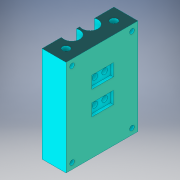
# Autodesk Inventor part: PowerPlugBlock
Saved by Autodesk Inventor 2019 (Build 230136000, 136)
## iProperties
Created: 2020-04-21
Part Number: PowerPlugBlock
Material: Generic
Document SubType Name: Modeling
Designer: james
Density: 1 g/cm^3
Appearance: Default(3)
Author: james
Autodesk Inventor part; units mm, degrees
ref_plane "YZ Plane" through (0, 0, 0) normal (1, 0, 0) x (0, 1, 0)
ref_plane "XZ Plane" through (0, 0, 0) normal (0, 1, 0) x (-1, 0, 0)
ref_plane "XY Plane" through (0, 0, 0) normal (0, 0, 1) x (1, 0, 0)
sketch "Sketch1" plane through (0, 0, 0) normal (0, 1, 0) x (-1, 0, 0)
  line L0 (7.4947, 23.2617) -> (-5.2053, 23.2617)
  line L1 (-5.2053, 23.2617) -> (-5.2053, -14.8383)
  line L2 (-5.2053, -14.8383) -> (7.4947, -14.8383)
  line L3 (7.4947, -14.8383) -> (7.4947, 23.2617)
  point P0 (0, 0)
  dimension "d0" = 38.1
  dimension "d1" = 12.7
  constraints: 8 end point, 2 parallel, 1 horizontal, 1 perpendicular
  measures "d0" distance of L0.end L1.end
  measures "d1" distance of L0.start L0.end
extrude "Extrusion1" add sketch "Sketch1" along normal blind 50.8
sketch "Sketch2" plane through (5.2053, 0, 23.2617) normal (1, 0, 0) x (0, 0, -1)
  line L0 (13.6294, 31.6) -> (25.1294, 31.6)
  line L1 (25.1294, 31.6) -> (25.1294, 38.1)
  line L2 (25.1294, 38.1) -> (13.6294, 38.1)
  line L3 (13.6294, 38.1) -> (13.6294, 31.6)
  line L4 (13.6294, 18.9) -> (25.1294, 18.9)
  line L5 (25.1294, 18.9) -> (25.1294, 25.4)
  line L6 (25.1294, 25.4) -> (13.6294, 25.4)
  line L7 (13.6294, 25.4) -> (13.6294, 18.9)
  line L8 (0, 0) -> (0, 50.8) projected
  line L9 (0, 0) -> (38.1, 0) projected
  line L10 (19.05, 56.7236) -> (19.05, -6.6913)
  point P0 (23.2617, 0)
  dimension "d4" = 11.5
  dimension "d5" = 0
  dimension "d6" = 0
  dimension "d8" = 25.4
  dimension "d9" = 12.7
  dimension "d10" = 6.5
  dimension "d11" = 6.5
  dimension "d47" = 19.05
  constraints: 18 end point, 4 parallel, 2 horizontal, 2 perpendicular, 1 vertical
  measures "d4" distance of L5.end L6.end
  measures "d5" distance between parallel lines of L7 L3
  measures "d6" distance between parallel lines of L5 L1
  measures "d8" distance between parallel lines of L9 L6
  measures "d9" distance between parallel lines of L6 L2
  measures "d10" distance of L2.end L0.start
  measures "d11" distance of L6.end L4.start
  measures "d47" distance between parallel lines of L8 L10
extrude "Extrusion2" cut sketch "Sketch2" against normal blind 1.524
sketch "Sketch3" plane through (3.6813, 0, 23.2617) normal (1, 0, 0) x (0, 0, -1)
  circle A0 centre (21.9544, 22.225) radius 1.5
  circle A1 centre (16.8044, 22.225) radius 1.5
  line L0 (13.6294, 25.4) -> (25.1294, 25.4) projected
  line L1 (13.6294, 18.9) -> (13.6294, 25.4) projected
  line L2 (25.1294, 25.4) -> (25.1294, 18.9) projected
  circle A2 centre (16.8044, 34.925) radius 1.5
  circle A3 centre (21.9544, 34.9504) radius 1.5
  line L3 (13.6294, 38.1) -> (25.1294, 38.1) projected
  point P0 (23.2617, 0)
  dimension "d15" = 3
  dimension "d16" = 3
  dimension "d17" = 3.175
  dimension "d18" = 3.175
  dimension "d19" = 3.175
  dimension "d20" = 3.175
  dimension "d21" = 3
  dimension "d22" = 3
  dimension "d23" = 3.175
  dimension "d24" = 3.1496
  dimension "d48" = 0
  dimension "d49" = 0
  constraints: 4 centre point
  measures "d15" diameter of A1
  measures "d16" diameter of A0
  measures "d17" distance from line of A1.centre L0
  measures "d18" distance from line of L1 A1.centre
  measures "d19" distance from line of A0.centre L0
  measures "d20" distance from line of L2 A0.centre
  measures "d21" diameter of A2
  measures "d22" diameter of A3
  measures "d23" distance from line of L3 A2.centre
  measures "d24" distance from line of L3 A3.centre
  measures "d48" horizontal distance of A1.centre A2.centre
  measures "d49" horizontal distance of A0.centre A3.centre
extrude "Extrusion3" cut sketch "Sketch3" against normal blind 41.3385
sketch "Sketch4" plane through (0, 0, 0) normal (0, -1, 0) x (1, 0, 0)
  line L0 (5.2053, -14.8383) -> (-7.4947, -14.8383) projected
  line L1 (5.2053, 23.2617) -> (5.2053, -14.8383) projected
  point P0 (0, 0)
  point P1 (-1.1447, 16.9117)
  point P2 (-1.1447, -8.4883)
  dimension "d27" = 25.4
  dimension "d28" = 6.35
  dimension "d29" = 6.35
  dimension "d30" = 0
  measures "d27" distance of point (-1.145, 16.912) point (-1.145, -8.488)
  measures "d28" distance from line of L0 point (-1.145, -8.488)
  measures "d29" distance from line of L1 point (-1.145, -8.488)
  measures "d30" horizontal distance of point (-1.145, -8.488) point (-1.145, 16.912)
hole "Hole1" at (-1.1447, 0, 16.9117) at (-1.1447, 0, -8.4883) direction (0, 1, 0) diameter 3.683 end through all thread size "10-24 UNC" class "2B" standard "ANSI Unified Screw Threads"
sketch "Sketch5" plane through (0, 0, 0) normal (0, -1, 0) x (1, 0, 0)
  circle A0 centre (-5.9707, 9.0377) radius 4.2329
  circle A1 centre (-5.9707, -0.6143) radius 4.2291
  line L0 (-7.4947, -14.8383) -> (-7.4947, 23.2617) projected
  line L1 (-7.4947, 23.2617) -> (5.2053, 23.2617) projected
  line L2 (5.2053, -14.8383) -> (-7.4947, -14.8383) projected
  point P0 (0, 0)
  dimension "d38" = 8.4658
  dimension "d39" = 8.4582
  dimension "d42" = 14.224
  dimension "d43" = 14.224
  dimension "d50" = 0
  dimension "d51" = 1.524
  constraints: 2 centre point
  measures "d38" diameter of A0
  measures "d39" diameter of A1
  measures "d42" distance from line of A0.centre L1
  measures "d43" distance from line of L2 A1.centre
  measures "d50" horizontal distance of A1.centre A0.centre
  measures "d51" distance from line of L0 A1.centre
extrude "Extrusion4" cut sketch "Sketch5" against normal blind 76.2
sketch "Sketch7" plane through (-7.4947, 0, 23.2617) normal (-1, 0, 0) x (0, 0, 1)
  line L0 (-38.1, 0) -> (-38.1, 50.8) projected
  line L1 (-38.1, 0) -> (-27.821, 0) projected
  line L2 (-38.1, 50.8) -> (-27.821, 50.8) projected
  line L3 (0, 0) -> (0, 50.8) projected
  point P0 (-23.2617, 0)
  point P1 (-34.925, 3.175)
  point P2 (-34.925, 47.625)
  point P3 (-3.175, 3.175)
  point P4 (-3.175, 47.625)
  dimension "d52" = 0
  dimension "d53" = 3.175
  dimension "d54" = 3.175
  dimension "d55" = 3.175
  dimension "d56" = 0
  dimension "d57" = 3.175
  dimension "d58" = 0
  dimension "d59" = 0
  measures "d52" horizontal distance of point (-34.925, 3.175) point (-34.925, 47.625)
  measures "d53" distance from line of L0 point (-34.925, 3.175)
  measures "d54" distance from line of L1 point (-34.925, 3.175)
  measures "d55" distance from line of L2 point (-34.925, 47.625)
  measures "d56" vertical distance of point (-3.175, 3.175) point (-34.925, 3.175)
  measures "d57" distance from line of L3 point (-3.175, 3.175)
  measures "d58" vertical distance of point (-3.175, 47.625) point (-34.925, 47.625)
  measures "d59" horizontal distance of point (-3.175, 3.175) point (-3.175, 47.625)
hole "Hole2" at (-7.4947, 3.175, -11.6633) at (-7.4947, 47.625, -11.6633) at (-7.4947, 3.175, 20.0867) at (-7.4947, 47.625, 20.0867) direction (1, 0, 0) diameter 2.4638 end through all
body "Solid1"
